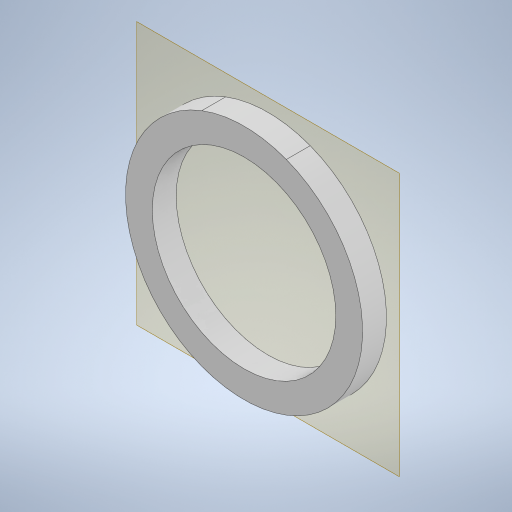
# Autodesk Inventor part: bearing-spacer-middle
Saved by Autodesk Inventor 2024 (Build 280153000, 153)
## iProperties
Created: 2024-04-07
Part Number: bearing-spacer-middle
Material: Generic
Document SubType Name: Modeling
Designer: MaartenGeorgesBuelen
Density: 1 g/cm^3
Appearance: Default
Author: MaartenGeorgesBuelen
## iProperties of the stored document bearing-spacer-middle_3DPrint.ipt
Created: 2024-04-07
Part Number: bearing-spacer-middle_3DPrint
Material: Generic
Document SubType Name: Modeling
Designer: MaartenGeorgesBuelen
Density: 1 g/cm^3
Appearance: Default
Author: MaartenGeorgesBuelen
Autodesk Inventor part; units mm, degrees
ref_plane "YZ Plane" through (0, 0, 0) normal (1, 0, 0) x (0, 1, 0)
ref_plane "Work Plane1" through (0, 0, 0) normal (0, 0, 1) x (1, 0, 0)
sketch "Sketch1" plane through (0, 0, 0) normal (0, 0, 1) x (1, 0, 0)
  circle A0 centre (0, 0) radius 19
  circle A1 centre (0, 0) radius 13.5
  circle A2 centre (0, 0) radius 19.2
  arc A3 (-8.918561, 23.355069) -> (8.918561, 23.355069) centre (0, 0) ccw
  arc A4 (-8.847213, 23.168229) -> (8.847213, 23.168229) centre (0, 0) ccw
  spline S0 degree 3 poles (-8.918561, 23.355069) (-5.800733, 24.545669) (-2.472604, 25.101169) (3.624662, 24.889005) (6.34449, 24.338026) (8.918561, 23.355069) knots 25.34476066 25.34476066 25.34476066 25.34476066 26.34598695 26.34598695 27.17143876 27.17143876 27.17143876 27.17143876
  arc A5 (-8.847213, 23.168229) -> (8.847213, 23.168229) centre (0, 0) ccw
  spline S1 degree 4 poles (-8.847213, 23.168229) (-4.622455, 24.781795) (0, 25.36818) (4.622456, 24.781802) (8.847213, 23.168229) knots 0 0 0 0 0 1 1 1 1 1
  point P0 (0, 0)
  point P1 (8.847213, 23.168229)
  dimension "d5" = 0.2
  dimension "d1" = 0.2
  dimension "d4" = 0.2
  constraints: 6 point on circle, 4 centre point, 1 concentric, 1 horizontal alignment, 9 other
  measures "d1" radial gap between concentric circles of A0 A2
  measures "d4" radial gap between concentric circles of A3 A4
ref_plane "Work Plane2" through (-19, -19, 5) normal (0, 0, 1) x (1, 0, 0)
ref_plane "Work Plane3" through (-19, -19, 5) normal (0, 0, 1) x (1, 0, 0)
sketch "Sketch1 outline for Extrusion2" plane through (0, 0, 0) normal (0, 0, 1) x (1, 0, 0)
  spline S0 degree 4 poles (-8.847213, 23.168229) (-4.622455, 24.781795) (0, 25.36818) (4.622456, 24.781802) (8.847213, 23.168229) knots 0 0 0 0 0 1 1 1 1 1
  arc A0 (-8.847213, 23.168229) -> (8.847213, 23.168229) centre (0, 0) ccw
  circle A1 centre (0, 0) radius 19.2
extrude "Extrusion2" add sketch "Sketch1 outline for Extrusion2" along normal up to surface (5 mm away)
body "Solid2"
